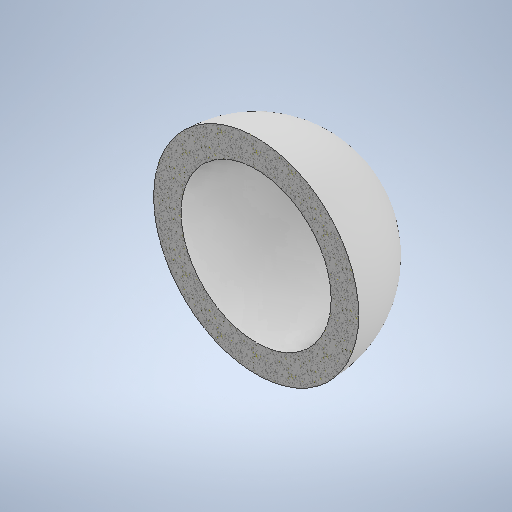
# Autodesk Inventor part: Peça2.esfera
Saved by Autodesk Inventor 2025.2 (Build 292293000, 293)
## iProperties
Created: 2025-03-26
Part Number: Peça2.esfera
Material: Genérico
Document SubType Name: Modeling
Designer: Formação
Density: 1 g/cm^3
Appearance: Padrão
Author: Formação
Autodesk Inventor part; units mm, degrees
ref_plane "YZ Plane" through (0, 0, 0) normal (1, 0, 0) x (0, 1, 0)
ref_plane "XZ Plane" through (0, 0, 0) normal (0, 1, 0) x (-1, 0, 0)
ref_plane "XY Plane" through (0, 0, 0) normal (0, 0, 1) x (1, 0, 0)
sketch "Esboço2" plane through (0, 0, 0) normal (0, 0, 1) x (1, 0, 0)
  circle A0 centre (6.5, 0) radius 0.5
  line L0 (0, -0.7) -> (0, 0.7) projected
  point P0 (0, 0)
  dimension "d8" = 6.5
  dimension "d9" = 1
  constraints: 1 centre point, 1 horizontal alignment
  measures "d8" distance of point (0, 0) A0.centre
  measures "d9" diameter of A0
revolve "Revolução2" [suppressed]
sketch "Esboço1" plane through (0, 0, 0) normal (0, 0, 1) x (1, 0, 0)
  line L0 (-7.5, 0.001) -> (7.5, -0.001) construction
  line L1 (0, -7.5) -> (0, 7.5) construction
  arc A0 (0, -7.5) -> (0, 7.5) centre (0, 0) ccw
  arc A1 (-0.0764, -5.4995) -> (0, 5.5) centre (0, 0) ccw
  line L2 (0, 7.5) -> (0, 5.5)
  line L3 (0, -5.5) -> (0, -7.5)
  line L4 (-10.5, 0) -> (10.5, 0) projected
  line L5 (0, -10.5) -> (0, 10.5) projected
  point P0 (0, 0)
  point P1 (0, 0)
  point P2 (0, 0)
  dimension "d0" = 15
  dimension "d1" = 15
  dimension "d2" = 2
  constraints: 8 end point, 6 point on circle, 4 coincident, 2 centre point, 2 collinear, 2 midpoint, 1 concentric, 1 vertical
  measures "d0" distance of L0.start L0.end
  measures "d1" distance of L1.start L1.end
  measures "d2" radial gap between concentric circles of A0 A1
revolve "Revolução1" add sketch "Esboço1" angle 360 mid plane about axis through (0, -10, 0) along (0, 1, 0) separate body contours L3 A1 L4 A0 | L4 A1 L2 A0
sketch "Esboço4" plane through (0, 0, 0) normal (0, 0, 1) x (1, 0, 0)
  circle A0 centre (0, 0) radius 1.5
  dimension "d11" = 3
  constraints: 2 coincident, 1 centre point
  measures "d11" diameter of A0
extrude "Extrusão1" cut sketch "Esboço4" along normal through all both and the other way through all
